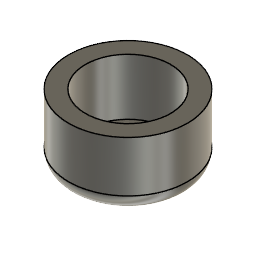
Cap 2 (Autodesk Fusion 360 design; units mm, degrees)
Autodesk Fusion 360 part; units mm, degrees
sketch "Sketch1" plane through (0, 0, 0) normal (0, 0, 1) x (1, 0, 0)
  circle A0 centre (0, 0) radius 7.55
  circle A1 centre (0, 0) radius 10.55
  dimension "d1" = 3
  dimension "d2" = 15.1
  constraint coincident A0.centre A1.centre
  measures "d2" diameter of A0
extrude "Extrude1" add sketch "Sketch1" along normal blind 10
extrude "Extrude2" add sketch "Sketch1" against normal blind 2 contours A0 | A1
fillet "Fillet1" radius 3 1 edges at (-9.8361, 3.815, -2)
